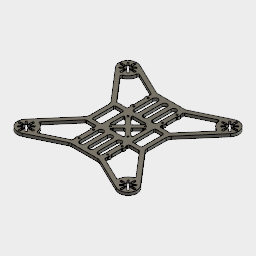
FPV Racing Chassis V7 (Autodesk Fusion 360 design; units mm, degrees)
Autodesk Fusion 360 part; units mm, degrees
note: some values were not read from the file. Chosen so that the rebuilt part matches the saved one: which face or edge a step refers to.
sketch "Frame Base Shape" plane through (0, 0, 0) normal (0, 1, 0) x (1, 0, 0)
  line L0 (18, -18) -> (-18, -18)
  line L1 (-18, -18) -> (-18, 18)
  line L2 (-18, 18) -> (18, 18)
  line L3 (18, 18) -> (18, -18)
  line L4 (18, -18) -> (-18, 18) construction
  line L5 (-18, -18) -> (18, 18) construction
  line L6 (15.25, -15.25) -> (-15.25, -15.25)
  line L7 (-15.25, -15.25) -> (-15.25, 15.25)
  line L8 (-15.25, 15.25) -> (15.25, 15.25)
  line L9 (15.25, 15.25) -> (15.25, -15.25)
  line L10 (15.25, -15.25) -> (-15.25, 15.25) construction
  line L11 (-15.25, -15.25) -> (15.25, 15.25) construction
  circle A0 centre (15.25, -15.25) radius 1.5
  circle A1 centre (-15.25, -15.25) radius 1.5
  circle A2 centre (-15.25, 15.25) radius 1.5
  circle A3 centre (15.25, 15.25) radius 1.5
  line L12 (0, 0) -> (88.3883, -88.3883) construction
  circle A4 centre (88.3883, -88.3883) radius 15.5
  line L13 (0, 0) -> (0, -75) construction
  line L14 (0, 0) -> (15.25, 0) construction
  line L15 (0, -75) -> (25, -75)
  line L16 (25, -75) -> (81.65, -102.347)
  line L17 (100.1384, -78.2797) -> (50, -20)
  line L18 (50, -20) -> (50, 0)
  line L19 (0, 75) -> (25, 75)
  line L20 (25, 75) -> (81.65, 102.347)
  circle A5 centre (88.3883, 88.3883) radius 15.5
  line L21 (100.1384, 78.2797) -> (50, 20)
  line L22 (50, 20) -> (50, 0)
  line L23 (0, 75) -> (-25, 75)
  line L24 (-25, 75) -> (-81.65, 102.347)
  circle A6 centre (-88.3883, 88.3883) radius 15.5
  line L25 (-100.1384, 78.2797) -> (-50, 20)
  line L26 (-50, 20) -> (-50, 0)
  line L27 (-50, -20) -> (-50, 0)
  line L28 (-100.1384, -78.2797) -> (-50, -20)
  circle A7 centre (-88.3883, -88.3883) radius 15.5
  line L29 (-25, -75) -> (-81.65, -102.347)
  line L30 (0, -75) -> (-25, -75)
  dimension "d1" = 36
  dimension "d2" = 30.5
  dimension "d3" = 3
  dimension "d4" = 125
  dimension "d5" = 31
  dimension "d6" = 75
  dimension "d7" = 25
  dimension "d8" = 50
  dimension "d9" = 20
  measures "d1" distance of L0.start L2.end
  measures "d2" distance of L6.start L8.end
  measures "d3" diameter of A3
  measures "d4" distance of L12.start L12.end
  measures "d5" diameter of A4
  measures "d6" distance of L12.start L13.end
  measures "d7" distance of L13.end L15.end
  measures "d8" distance of L12.start L18
  measures "d9" distance of L17.end L18.end
extrude "Chassis Base" add sketch "Frame Base Shape" along normal blind 5 contours L0 L1 L2 L3 | L6 L7 L8 L9 A0 A1 A2 A3 | A4 | A4 L15 L16 L17 L18 L19 L20 A5 L21 L22 L23 L24 A6 L25 L26 L27 L28 A7 L29 L30 | A5 | A7 | A6
sketch "Motor Mount" plane through (0, 0, 0) normal (0, 1, 0) x (1, 0, 0)
  circle A0 centre (88.3883, -88.3883) radius 5
  line L0 (86.8883, -76.3883) -> (86.8883, -81.3883)
  arc A1 (86.8883, -81.3883) -> (89.8883, -81.3883) centre (88.3883, -81.3883) ccw
  line L1 (89.8883, -81.3883) -> (89.8883, -76.3883)
  arc A2 (89.8883, -76.3883) -> (86.8883, -76.3883) centre (88.3883, -76.3883) ccw
  line L2 (88.3883, -76.3883) -> (88.3883, -81.3883) construction
  line L3 (94.5755, -80.4334) -> (91.04, -83.9689)
  arc A3 (91.04, -83.9689) -> (92.8078, -85.7367) centre (91.9239, -84.8528) ccw
  line L4 (92.8078, -85.7367) -> (96.3433, -82.2012)
  arc A4 (96.3433, -82.2012) -> (94.5755, -80.4334) centre (95.4594, -81.3173) ccw
  line L5 (95.4594, -81.3173) -> (91.9239, -84.8528) construction
  arc A5 (76.3883, -86.8883) -> (76.3883, -89.8883) centre (76.3883, -88.3883) ccw
  line L6 (81.3883, -86.8883) -> (76.3883, -86.8883)
  arc A6 (81.3883, -89.8883) -> (81.3883, -86.8883) centre (81.3883, -88.3883) ccw
  line L7 (76.3883, -89.8883) -> (81.3883, -89.8883)
  arc A7 (83.9689, -85.7367) -> (85.7367, -83.9689) centre (84.8528, -84.8528) ccw
  line L8 (85.7367, -83.9689) -> (82.2012, -80.4334)
  line L9 (80.4334, -82.2012) -> (83.9689, -85.7367)
  arc A8 (82.2012, -80.4334) -> (80.4334, -82.2012) centre (81.3173, -81.3173) ccw
  arc A9 (86.8883, -100.3883) -> (89.8883, -100.3883) centre (88.3883, -100.3883) ccw
  line L10 (86.8883, -95.3883) -> (86.8883, -100.3883)
  arc A10 (89.8883, -95.3883) -> (86.8883, -95.3883) centre (88.3883, -95.3883) ccw
  line L11 (89.8883, -100.3883) -> (89.8883, -95.3883)
  arc A11 (85.7367, -92.8078) -> (83.9689, -91.04) centre (84.8528, -91.9239) ccw
  line L12 (83.9689, -91.04) -> (80.4334, -94.5755)
  line L13 (82.2012, -96.3433) -> (85.7367, -92.8078)
  arc A12 (80.4334, -94.5755) -> (82.2012, -96.3433) centre (81.3173, -95.4594) ccw
  arc A13 (100.3883, -89.8883) -> (100.3883, -86.8883) centre (100.3883, -88.3883) ccw
  line L14 (95.3883, -89.8883) -> (100.3883, -89.8883)
  arc A14 (95.3883, -86.8883) -> (95.3883, -89.8883) centre (95.3883, -88.3883) ccw
  line L15 (100.3883, -86.8883) -> (95.3883, -86.8883)
  arc A15 (92.8078, -91.04) -> (91.04, -92.8078) centre (91.9239, -91.9239) ccw
  line L16 (91.04, -92.8078) -> (94.5755, -96.3433)
  line L17 (96.3433, -94.5755) -> (92.8078, -91.04)
  arc A16 (94.5755, -96.3433) -> (96.3433, -94.5755) centre (95.4594, -95.4594) ccw
  point P0 (88.3883, -88.3883)
  dimension "d12" = 10
  dimension "d13" = 1.5
  dimension "d14" = 7
  dimension "d15" = 12
  dimension "d16" = 1.25
  dimension "d17" = 5
  dimension "d18" = 10
  dimension "d19" = 45
  dimension "d21" = 360
  measures "d12" diameter of A0
  measures "d13" radius of A2
  measures "d14" distance of P0 A1.centre
  measures "d15" distance of P0 A2.centre
  measures "d16" radius of A3
  measures "d17" distance of P0 A3.centre
  measures "d18" distance of P0 A4.centre
  measures "d19" angle of L2 L5
extrude "Motor Mount (1)" cut sketch "Motor Mount" along normal through all
mirror "Mirror1" about plane through (0, 0, 0) normal (0, 0, 1) of "Motor Mount (1)"
mirror "Mirror2" about plane through (0, 0, 0) normal (1, 0, 0) of "Motor Mount (1)", "Mirror1"
sketch "Frame Cutouts" plane through (0, 0, 0) normal (0, 1, 0) x (1, 0, 0)
  circle A0 centre (15.25, 15.25) radius 4.5
  circle A1 centre (15.25, -15.25) radius 4.5
  circle A2 centre (-15.25, -15.25) radius 4.5
  circle A3 centre (-15.25, 15.25) radius 4.5
  circle A4 centre (15.25, 15.25) radius 1.5
  line L0 (-15.25, 15.25) -> (15.25, -15.25) construction
  line L1 (-15.25, -15.25) -> (15.25, 15.25) construction
  line L2 (19.75, 15.25) -> (19.75, -15.25)
  line L3 (15.25, -19.75) -> (-15.25, -19.75)
  line L4 (-19.75, -15.25) -> (-19.75, 15.25)
  line L5 (-15.25, 19.75) -> (15.25, 19.75)
  line L6 (-12.7751, -17.7249) -> (17.7249, 12.7751)
  line L7 (-17.7249, -12.7751) -> (12.7751, 17.7249)
  line L8 (-17.7249, 12.7751) -> (12.7751, -17.7249)
  line L9 (-12.7751, 17.7249) -> (17.7249, -12.7751)
  line L10 (43, -19.75) -> (26.75, -19.75)
  line L11 (26.75, -19.75) -> (26.75, 19.75)
  line L12 (26.75, 19.75) -> (43, 19.75)
  line L13 (43, 19.75) -> (43, -19.75)
  line L14 (43, -19.75) -> (26.75, 19.75) construction
  line L15 (26.75, -19.75) -> (43, 19.75) construction
  line L16 (50, -20) -> (50, 20)
  line L17 (0, 0) -> (0, 13.5162) construction
  line L18 (0, 0) -> (12.9723, 0) construction
  line L19 (-26.75, 19.75) -> (-43, 19.75)
  line L20 (-26.75, -19.75) -> (-26.75, 19.75)
  line L21 (-43, 19.75) -> (-43, -19.75)
  line L22 (-43, -19.75) -> (-26.75, -19.75)
  line L23 (100.1384, -78.2797) -> (50, -20)
  line L24 (25, -75) -> (81.65, -102.347)
  arc A5 (81.65, -102.347) -> (100.1384, -78.2797) centre (88.3883, -88.3883) ccw
  line L25 (28.0431, -68.6961) -> (84.6931, -96.0431)
  arc A6 (84.6931, -96.0431) -> (94.8319, -82.8449) centre (88.3883, -88.3883) ccw
  line L26 (94.8319, -82.8449) -> (44.6935, -24.5652)
  circle A7 centre (25, -60) radius 1.5
  circle A8 centre (25, -35) radius 1.5
  line L27 (-25, -75) -> (25, -75)
  circle A9 centre (25, -60) radius 4.5
  circle A10 centre (25, -35) radius 4.5
  line L28 (28.0431, -68.6961) -> (28.0431, -26.75)
  line L29 (28.0431, -26.75) -> (46.5731, -26.75)
  circle A11 centre (88.3883, -88.3883) radius 17.5
  line L30 (-20.5, -31.25) -> (-20.5, -63.5)
  arc A12 (-20.5, -63.5) -> (-11.5, -63.5) centre (-16, -63.5) ccw
  line L31 (-11.5, -63.5) -> (-11.5, -31.25)
  arc A13 (-11.5, -31.25) -> (-20.5, -31.25) centre (-16, -31.25) ccw
  line L32 (-16, -31.25) -> (-16, -63.5) construction
  line L33 (-4.5, -31.25) -> (-4.5, -63.5)
  arc A14 (-4.5, -63.5) -> (4.5, -63.5) centre (0, -63.5) ccw
  line L34 (4.5, -63.5) -> (4.5, -31.25)
  arc A15 (4.5, -31.25) -> (-4.5, -31.25) centre (0, -31.25) ccw
  line L35 (0, -31.25) -> (0, -63.5) construction
  line L36 (11.5, -31.25) -> (11.5, -63.5)
  arc A16 (11.5, -63.5) -> (20.5, -63.5) centre (16, -63.5) ccw
  line L37 (20.5, -63.5) -> (20.5, -31.25)
  arc A17 (20.5, -31.25) -> (11.5, -31.25) centre (16, -31.25) ccw
  line L38 (16, -31.25) -> (16, -63.5) construction
  arc A18 (-11.5, 63.5) -> (-20.5, 63.5) centre (-16, 63.5) ccw
  line L39 (-11.5, 63.5) -> (-11.5, 31.25)
  line L40 (-20.5, 31.25) -> (-20.5, 63.5)
  arc A19 (-20.5, 31.25) -> (-11.5, 31.25) centre (-16, 31.25) ccw
  line L41 (-4.5, 31.25) -> (-4.5, 63.5)
  arc A20 (4.5, 63.5) -> (-4.5, 63.5) centre (0, 63.5) ccw
  arc A21 (-4.5, 31.25) -> (4.5, 31.25) centre (0, 31.25) ccw
  line L42 (4.5, 63.5) -> (4.5, 31.25)
  line L43 (20.5, 63.5) -> (20.5, 31.25)
  arc A22 (11.5, 31.25) -> (20.5, 31.25) centre (16, 31.25) ccw
  arc A23 (20.5, 63.5) -> (11.5, 63.5) centre (16, 63.5) ccw
  line L44 (11.5, 31.25) -> (11.5, 63.5)
  circle A24 centre (25, 35) radius 4.5
  circle A25 centre (25, 35) radius 1.5
  circle A26 centre (25, 60) radius 1.5
  circle A27 centre (25, 60) radius 4.5
  line L45 (28.0431, 68.6961) -> (28.0431, 26.75)
  line L46 (28.0431, 68.6961) -> (84.6931, 96.0431)
  line L47 (28.0431, 26.75) -> (46.5731, 26.75)
  line L48 (94.8319, 82.8449) -> (44.6935, 24.5652)
  circle A28 centre (88.3883, 88.3883) radius 17.5
  arc A29 (94.8319, 82.8449) -> (84.6931, 96.0431) centre (88.3883, 88.3883) ccw
  circle A30 centre (-25, 60) radius 4.5
  circle A31 centre (-25, 60) radius 1.5
  circle A32 centre (-25, 35) radius 4.5
  circle A33 centre (-25, 35) radius 1.5
  line L49 (-28.0431, 68.6961) -> (-28.0431, 26.75)
  line L50 (-28.0431, 26.75) -> (-46.5731, 26.75)
  line L51 (-94.8319, 82.8449) -> (-44.6935, 24.5652)
  line L52 (-28.0431, 68.6961) -> (-84.6931, 96.0431)
  circle A34 centre (-88.3883, 88.3883) radius 17.5
  arc A35 (-84.6931, 96.0431) -> (-94.8319, 82.8449) centre (-88.3883, 88.3883) ccw
  line L53 (-28.0431, -26.75) -> (-46.5731, -26.75)
  line L54 (-94.8319, -82.8449) -> (-44.6935, -24.5652)
  line L55 (-28.0431, -68.6961) -> (-28.0431, -26.75)
  line L56 (-28.0431, -68.6961) -> (-84.6931, -96.0431)
  circle A36 centre (-88.3883, -88.3883) radius 17.5
  arc A37 (-94.8319, -82.8449) -> (-84.6931, -96.0431) centre (-88.3883, -88.3883) ccw
  circle A38 centre (-25, -35) radius 1.5
  circle A39 centre (-25, -35) radius 4.5
  circle A40 centre (-25, -60) radius 1.5
  circle A41 centre (-25, -60) radius 4.5
  point P0 (15.25, 15.25)
  point P1 (15.25, -15.25)
  point P2 (-15.25, -15.25)
  point P3 (-15.25, 15.25)
  point P4 (34.875, 0)
  dimension "d25" = 3
  dimension "d26" = 3.5
  dimension "d27" = 3.5
  dimension "d28" = 3.5
  dimension "d29" = 3.5
  dimension "d30" = 7
  dimension "d31" = 7
  dimension "d32" = 7
  dimension "d33" = 3
  dimension "d34" = 25
  dimension "d35" = 25
  dimension "d36" = 15
  dimension "d37" = 3
  dimension "d38" = 7
  dimension "d39" = 35
  dimension "d40" = 4.5
  dimension "d41" = 7
  dimension "d42" = 7
  dimension "d43" = 11.5
  dimension "d44" = 11.5
  measures "d25" distance of A0 A4
  measures "d30" distance of L13 L16
  measures "d31" distance of L2 L11
  measures "d33" diameter of A8
  measures "d34" distance of L17.start A8.centre
  measures "d35" distance of A7.centre A8.centre
  measures "d36" distance of A7.centre L27
  measures "d37" distance of A8 A10
  measures "d38" distance of L10 L29
  measures "d39" diameter of A11
  measures "d40" radius of A15
  measures "d41" distance of L31 L33
  measures "d42" distance of L34 L36
  measures "d43" distance of L3 A15.centre
  measures "d44" distance of L27 A14.centre
extrude "Extrude3" cut sketch "Frame Cutouts" along normal through all contours A0 A1 L2 L6 L9 | A0 A3 L5 L7 L9 | A1 A2 L3 L6 L8 | A2 A3 L4 L7 L8 | L10 L11 L12 L13 | L19 L20 L21 L22 | L25 L26 A9 A10 L28 L29 A11 | L36 A16 L37 A17 | A7 | A8 | L30 A12 L31 A13 | L53 L54 L55 L56 A36 A39 A41 | L33 A14 L34 A15 | A18 L39 L40 A19 | A30 A32 L49 L50 L51 L52 A34 | L41 A20 A21 L42 | L43 A22 A23 L44 | A24 A27 L45 L46 L47 L48 A28 | A25 | A26 | A31 | A33 | A38 | A40
fillet "Fillet1" radius 2 56 edges at (-28.0431, 2.5, 38.315) (-28.0431, 2.5, 31.685) (-28.0431, 2.5, 26.75) (-46.5731, 2.5, 26.75) (-84.8556, 2.5, 71.2486) (-70.9172, 2.5, 89.393) (-28.0431, 2.5, 68.6961) (-28.0431, 2.5, 63.315) (-28.0431, 2.5, 56.685) (-43, 2.5, -19.75) (-26.75, 2.5, -19.75) (-43, 2.5, 19.75) (-26.75, 2.5, 19.75) (70.9172, 2.5, 89.393) (84.8556, 2.5, 71.2486) (46.5731, 2.5, 26.75) (28.0431, 2.5, 26.75) (28.0431, 2.5, 31.685) (28.0431, 2.5, 38.315) (28.0431, 2.5, 56.685) (28.0431, 2.5, 63.315) (28.0431, 2.5, 68.6961) (10.7751, 2.5, 15.7249) (0, 2.5, 4.9497) (-10.7751, 2.5, 15.7249) (-15.7249, 2.5, -10.7751) (-15.7249, 2.5, 10.7751) (-4.9497, 2.5, 0) (-28.0431, 2.5, -56.685) (-28.0431, 2.5, -63.315) (-28.0431, 2.5, -68.6961) (-70.9172, 2.5, -89.393) (-84.8556, 2.5, -71.2486) (-46.5731, 2.5, -26.75) (-28.0431, 2.5, -26.75) (-28.0431, 2.5, -31.685) (-28.0431, 2.5, -38.315) (15.7249, 2.5, -10.7751) (4.9497, 2.5, 0) (15.7249, 2.5, 10.7751) (10.7751, 2.5, -15.7249) (-10.7751, 2.5, -15.7249) (0, 2.5, -4.9497) (26.75, 2.5, 19.75) (43, 2.5, 19.75) (43, 2.5, -19.75) (26.75, 2.5, -19.75) (28.0431, 2.5, -63.315) (28.0431, 2.5, -56.685) (28.0431, 2.5, -38.315) (28.0431, 2.5, -31.685) (28.0431, 2.5, -26.75) (46.5731, 2.5, -26.75) (84.8556, 2.5, -71.2486) (70.9172, 2.5, -89.393) (28.0431, 2.5, -68.6961)
fillet "Fillet2" radius 1 8 edges at (15.25, 2.5, -19.75) (-15.25, 2.5, -19.75) (-19.75, 2.5, -15.25) (-19.75, 2.5, 15.25) (-15.25, 2.5, 19.75) (15.25, 2.5, 19.75) (19.75, 2.5, 15.25) (19.75, 2.5, -15.25)
fillet "Fillet3" radius 10 8 edges at (50, 2.5, -20) (50, 2.5, 20) (-50, 2.5, -20) (-50, 2.5, 20) (-25, 2.5, -75) (25, 2.5, -75) (-25, 2.5, 75) (25, 2.5, 75)
equation "d43 = 7 mm + d40"
equation "d44 = d43"
